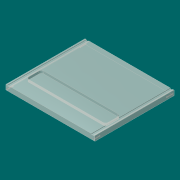
# Autodesk Inventor part: topBottom
Saved by Autodesk Inventor 2016 (Build 200138000, 138)
## iProperties
Created: 2015-10-13
Part Number: topBottom
Material: PC/ABS Plastic
Document SubType Name: Modeling
Designer: Sawaiz
Density: 0.357273 g/cm^3
Appearance: Clear
Author: Sawaiz
Autodesk Inventor part; units mm, degrees
ref_plane "YZ Plane" through (0, 0, 0) normal (1, 0, 0) x (0, 1, 0)
ref_plane "XZ Plane" through (0, 0, 0) normal (0, 1, 0) x (-1, 0, 0)
ref_plane "XY Plane" through (0, 0, 0) normal (0, 0, 1) x (1, 0, 0)
sketch "Sketch1" plane through (0, 0, 0) normal (0, 0, 1) x (1, 0, 0)
  line L0 (-50.8, -57.15) -> (50.8, -57.15)
  line L1 (50.8, -57.15) -> (50.8, 57.15)
  line L2 (50.8, 57.15) -> (-50.8, 57.15)
  line L3 (-50.8, 57.15) -> (-50.8, -57.15)
  line L4 (-50.8, -57.15) -> (50.8, 57.15) construction
  line L5 (50.8, -57.15) -> (-50.8, 57.15) construction
  point P0 (0, 0)
  dimension "d0" = 101.6
  dimension "d1" = 114.3
  constraints: 12 end point, 2 midpoint, 2 parallel, 1 horizontal, 1 perpendicular
  measures "d0" distance of L2.end L1.end
  measures "d1" distance of L1.end L0.end
extrude "Extrusion1" add sketch "Sketch1" along normal blind 6.35
sketch "Sketch7" plane through (50.8, -57.15, 0) normal (1, 0, 0) x (0, 0, -1)
  line L0 (0, 0) -> (0, 114.3) projected
  line L1 (0, 114.3) -> (-6.35, 114.3) projected
  line L2 (-6.35, 0) -> (-6.35, 114.3) projected
  line L3 (0, 0) -> (-6.35, 0) projected
  line L4 (-1.5875, 0) -> (-1.5875, 114.3)
  point P0 (0, 57.15)
  point P1 (-1.5875, 1.5875)
  point P2 (-1.5875, 112.7125)
  dimension "d46" = 1.5875
  dimension "d47" = 1.5875
  dimension "d48" = 1.5875
  constraints: 4 point on line, 2 end point, 1 perpendicular
  measures "d46" distance between parallel lines of L0 L4
  measures "d47" distance from line of L1 point (-1.588, 112.713)
  measures "d48" distance from line of L3 point (-1.587, 1.587)
hole "Hole3" at (50.8, -55.5625, 1.5875) at (50.8, 55.5625, 1.5875) direction (-1, 0, 0) diameter 1.181 depth 7.938 tip angle 118 thread size "0-80 UNF" class "2B" standard "ANSI Unified Screw Threads"
mirror "Mirror3" about plane through (0, 0, 0) normal (1, 0, 0) of "Hole3"
sketch "Sketch8" plane through (0, 0, 6.35) normal (0, 0, 1) x (1, 0, 0)
  line L0 (-50.8, -57.15) -> (50.8, -57.15) projected
  line L1 (50.8, -57.15) -> (50.8, 57.15) projected
  line L2 (50.8, 57.15) -> (-50.8, 57.15) projected
  line L3 (-50.8, 57.15) -> (-50.8, -57.15) projected
  line L4 (30.8, -50.8) -> (11.75, -50.8)
  line L5 (11.75, -50.8) -> (11.75, 50.8)
  line L6 (11.75, 50.8) -> (30.8, 50.8)
  line L7 (30.8, 50.8) -> (30.8, -50.8)
  point P0 (0, 0)
  dimension "d59" = 20
  dimension "d60" = 19.05
  dimension "d63" = 6.35
  dimension "d64" = 6.35
  constraints: 8 end point, 2 parallel, 1 horizontal, 1 perpendicular
  measures "d59" distance between parallel lines of L1 L7
  measures "d60" distance between parallel lines of L5 L7
  measures "d63" distance between parallel lines of L0 L4
  measures "d64" distance between parallel lines of L2 L6
extrude "Extrusion4" cut sketch "Sketch8" against normal blind 3.175 contours L4 L5 L6 L7
sketch "Sketch9" plane through (0, 0, 6.35) normal (0, 0, 1) x (1, 0, 0)
  line L0 (11.75, 50.8) -> (30.8, 50.8) projected
  line L1 (30.8, 50.8) -> (30.8, -50.8) projected
  line L2 (30.8, -50.8) -> (11.75, -50.8) projected
  line L3 (11.75, -50.8) -> (11.75, 50.8) projected
  line L4 (-50.8, -57.15) -> (50.8, -57.15) projected
  line L5 (50.8, -57.15) -> (50.8, 57.15) projected
  line L6 (50.8, 57.15) -> (-50.8, 57.15) projected
  line L7 (-50.8, 57.15) -> (-50.8, -57.15) projected
  line L8 (50.8, -57.15) -> (50.8, 57.15) projected
  line L9 (50.8, 52.3875) -> (-50.8, 52.3875)
  line L10 (-50.8, 52.3875) -> (-50.8, 55.5625)
  line L11 (-50.8, 55.5625) -> (50.8, 55.5625)
  line L12 (50.8, 55.5625) -> (50.8, 52.3875)
  point P0 (0, 0)
  dimension "d65" = 1.5875
  dimension "d66" = 3.175
  constraints: 8 end point, 2 parallel, 2 point on line, 1 horizontal, 1 perpendicular
  measures "d65" distance between parallel lines of L6 L11
  measures "d66" distance between parallel lines of L9 L11
extrude "Extrusion5" cut sketch "Sketch9" against normal blind 0.9525 contours L7 L11 L5 L9
mirror "Mirror4" about plane through (0, 0, 0) normal (0, 1, 0) of "Extrusion5"
fillet "Fillet1" radius 3.175 4 edges at (11.75, -50.8, 4.7625) (30.8, -50.8, 4.7625) (30.8, 50.8, 4.7625) (11.75, 50.8, 4.7625)
equation "\"d0\" = depth"
equation "\"d1\" = width + 2 * acrylicThickness"
equation "\"d2\" = acrylicThickness"
equation "\"d46\" = 0.25 * acrylicThickness"
equation "\"d47\" = 0.25 * acrylicThickness"
equation "\"d48\" = 0.25 * acrylicThickness"
equation "\"d59\" = aerogelThickness"
equation "\"d60\" = mirrorGroove"
equation "\"d63\" = acrylicThickness"
equation "\"d64\" = acrylicThickness"
equation "\"d61\" = 0.5 * acrylicThickness"
equation "\"d65\" = 0.5 * acrylicThickness - 0.5 * oRingWidth"
equation "\"d66\" = oRingWidth"
equation "\"d69\" = mirrorGrooveMill"
equation "\"acrylicThickness\" = 6.35"
equation "\"width\" = 101.6"
equation "\"depth\" = 101.6"
equation "\"aerogelThickness\" = 20"
equation "\"oRingWidth\" = 3.175"
equation "\"mirrorGroove\" = 19.05"
equation "\"mirrorGrooveMill\" = 3.175"
equation "\"height\" = 101.6"
equation "\"mirrorAngle\" = 5deg"
equation "\"detectorWidth\" = 52"
equation "\"detectorHeight\" = 52"
equation "\"mirrorThickness\" = 3"
equation "\"fresnelThickness\" = 0.1"
equation "\"focalLength\" = 76.2"
equation "\"ior\" = 1.49"
equation "\"centerThickness\" = 1.524"
equation "\"fresnelAngle\" = 90deg"
equation "\"fresnelEffectiveDiameter\" = 76.2"
equation "\"mirrorSuppourtWidth\" = 38.1"
equation "\"backGrooveBit\" = 4.8006"
equation "\"sensorHolderWidth\" = 88.9"
equation "\"sensorHolderHeight\" = 88.9"
equation "\"sensorHolderSensorHeight\" = 53.975"
equation "\"sensorHolderSensorWidth\" = 53.975"
equation "\"sensorHolderORingID\" = 203.2"
equation "\"sensorHolderFlushORingID\" = 304.8"
equation "\"frontBackORingID\" = 419.1"
equation "\"backMirrorGroove\" = 6.35"
equation "\"fresnelChamfer\" = 6.35"
equation "\"fresnelMirrorChamfer\" = 6.35"
equation "\"detectorOpeningHeight\" = 76.2"
equation "\"detectorOpeningWidth\" = 76.2"
body "Solid1"
